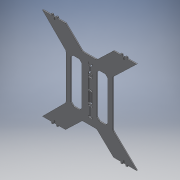
# Autodesk Inventor part: Z stage_brace
Saved by Autodesk Inventor 2019 (Build 230136000, 136)
## iProperties
Created: 2020-03-07
Part Number: Z stage_brace
Material: Generic
Document SubType Name: Modeling
Designer: Vijay
Density: 1 g/cm^3
Appearance: Default
Author: Vijay
Autodesk Inventor part; units mm, degrees
ref_plane "YZ Plane" through (0, 0, 0) normal (1, 0, 0) x (0, 1, 0)
ref_plane "XZ Plane" through (0, 0, 0) normal (0, 1, 0) x (-1, 0, 0)
ref_plane "XY Plane" through (0, 0, 0) normal (0, 0, 1) x (1, 0, 0)
sketch "Sketch1" plane through (0, 0, 0) normal (0, 0, 1) x (1, 0, 0)
  line L0 (428.5825, 0) -> (20, 0) projected
  line L1 (20, -400) -> (428.5825, -400) projected
  line L2 (328.5883, 0) -> (224.2968, -100)
  line L3 (224.2968, -100) -> (120, 0)
  line L4 (328.5825, -400) -> (224.2968, -300)
  line L5 (224.2968, -300) -> (120, -400)
  line L6 (224.2968, 24.0361) -> (224.2968, -493.2268) construction
  line L7 (428.5825, 0) -> (328.5883, 0)
  line L8 (120, 0) -> (19.9984, 0)
  line L9 (20, -400) -> (120, -400)
  line L10 (328.5825, -400) -> (428.5824, -400)
  line L11 (19.9984, 0) -> (122.1697, -102.1708)
  line L12 (122.1697, -102.1708) -> (122.1708, -297.8287)
  line L13 (122.1708, -297.8287) -> (20, -400)
  line L14 (428.5825, 0) -> (324.2968, -100.0061)
  line L15 (324.2968, -100.0061) -> (324.2968, -300)
  line L16 (324.2968, -300) -> (428.5824, -400)
  line L17 (255.5843, -70) -> (193.0078, -70)
  line L18 (255.5825, -330) -> (193.0078, -330)
  line L19 (20, -400) -> (20, -400)
  point P0 (0, 0)
  dimension "d1" = 100
  dimension "d2" = 100
  dimension "d3" = 100
  dimension "d4" = 104.2915
  dimension "d5" = 100
  dimension "d6" = 100
  dimension "d7" = 100
  dimension "d8" = 70
  dimension "d9" = 70
  constraints: 36 end point, 7 point on line, 4 equal length, 4 horizontal, 4 parallel, 3 perpendicular, 2 collinear, 2 vertical
  measures "d1" distance of L4.start L1.end
  measures "d2" distance of L5.end L1.start
  measures "d3" distance of L3.end L0.end
  measures "d4" distance from line of L6 L2.start
  measures "d5" distance from line of L0 L2.end
  measures "d6" distance from line of L1 L4.end
  measures "d7" distance between parallel lines of L6 L15
  measures "d8" distance between parallel lines of L0 L17
  measures "d9" distance between parallel lines of L1 L18
extrude "Extrusion1" add sketch "Sketch1" against normal blind 4 contours L14 L15 L16 L1 L4 L5 L13 L12 L11 L0 L3 L2 | L2 L3 L17 | L18 L5 L4
fillet "Fillet1" radius 10 8 edges at (324.2968, -100.0061, -2) (324.2968, -300, -2) (255.5825, -330, -2) (193.0078, -330, -2) (122.1708, -297.8287, -2) (122.1697, -102.1708, -2) (193.0078, -70, -2) (255.5843, -70, -2)
sketch "Sketch2" plane through (0, 0, -4) normal (0, 0, -1) x (-1, 0, 0)
  line L0 (-235.5222, -304.8491) -> (-235.5222, -94.8768) construction
  line L1 (-235.5222, -94.8768) -> (-217.757, -94.8768) construction
  line L2 (-217.757, -94.8768) -> (-217.757, -304.8491) construction
  line L3 (-217.757, -304.8491) -> (-235.5222, -304.8491) construction
  line L4 (-217.757, -297.1164) -> (-224.4247, -297.1164)
  line L5 (-224.4247, -297.1164) -> (-224.4247, -260.8142)
  line L6 (-224.4247, -260.8142) -> (-217.757, -260.8142)
  line L7 (-217.757, -260.8142) -> (-217.757, -255.0571)
  line L8 (-217.757, -255.0571) -> (-235.5222, -255.0571)
  line L9 (-235.5222, -255.0571) -> (-235.5222, -260.8142)
  line L10 (-235.5222, -260.8142) -> (-228.8545, -260.8142)
  line L11 (-228.8545, -260.8142) -> (-228.8545, -297.1164)
  line L12 (-228.8545, -297.1164) -> (-235.5222, -297.1164)
  line L13 (-235.5222, -297.1164) -> (-235.5222, -302.8735)
  line L14 (-235.5222, -302.8735) -> (-217.757, -302.8735)
  line L15 (-217.757, -302.8735) -> (-217.757, -297.1164)
  line L16 (-224.4247, -205.5429) -> (-228.8545, -205.5429)
  line L17 (-228.8545, -205.5429) -> (-228.8545, -245.3487)
  line L18 (-228.8545, -245.3487) -> (-229.7651, -245.3487)
  spline S0 degree 2 poles (-229.7651, -245.3487) (-230.3053, -245.3487) (-231.1079, -244.7777) (-231.1079, -244.1603) knots 0 0 0 1 2 2 2
  line L19 (-231.1079, -244.1603) -> (-231.1079, -205.4966)
  line L20 (-231.1079, -205.4966) -> (-235.5222, -205.4966)
  line L21 (-235.5222, -205.4966) -> (-235.5222, -247.17)
  spline S1 degree 2 poles (-235.5222, -247.17) (-235.5222, -249.2383) (-233.3923, -251.1058) (-231.5555, -251.1058) knots 0 0 0 1 2 2 2
  line L22 (-231.5555, -251.1058) -> (-221.7237, -251.1058)
  spline S2 degree 2 poles (-221.7237, -251.1058) (-219.887, -251.1058) (-217.757, -249.2383) (-217.757, -247.17) knots 0 0 0 1 2 2 2
  line L23 (-217.757, -247.17) -> (-217.757, -205.4966)
  line L24 (-217.757, -205.4966) -> (-222.1867, -205.4966)
  line L25 (-222.1867, -205.4966) -> (-222.1867, -244.1603)
  spline S3 degree 2 poles (-222.1867, -244.1603) (-222.1867, -244.7777) (-222.9739, -245.3487) (-223.5141, -245.3487) knots 0 0 0 1 2 2 2
  line L26 (-223.5141, -245.3487) -> (-224.4247, -245.3487)
  line L27 (-224.4247, -245.3487) -> (-224.4247, -205.5429)
  line L28 (-235.5222, -201.5453) -> (-221.7237, -201.5453)
  spline S4 degree 2 poles (-221.7237, -201.5453) (-219.887, -201.5453) (-217.757, -199.6778) (-217.757, -197.6095) knots 0 0 0 1 2 2 2
  line L29 (-217.757, -197.6095) -> (-217.757, -155.9361)
  line L30 (-217.757, -155.9361) -> (-222.1867, -155.9361)
  line L31 (-222.1867, -155.9361) -> (-222.1867, -194.5998)
  spline S5 degree 2 poles (-222.1867, -194.5998) (-222.1867, -195.2172) (-222.9739, -195.7882) (-223.5141, -195.7882) knots 0 0 0 1 2 2 2
  line L32 (-223.5141, -195.7882) -> (-235.5222, -195.7882)
  line L33 (-235.5222, -195.7882) -> (-235.5222, -201.5453)
  line L34 (-217.757, -146.1814) -> (-235.5222, -146.1814)
  line L35 (-235.5222, -146.1814) -> (-235.5222, -151.9848)
  line L36 (-235.5222, -151.9848) -> (-217.757, -151.9848)
  line L37 (-217.757, -151.9848) -> (-217.757, -146.1814)
  line L38 (-235.5222, -95.7103) -> (-235.5222, -103.3041)
  line L39 (-235.5222, -103.3041) -> (-228.8545, -111.4227)
  line L40 (-228.8545, -111.4227) -> (-228.8545, -127.6599)
  line L41 (-228.8545, -127.6599) -> (-235.5222, -135.7785)
  line L42 (-235.5222, -135.7785) -> (-235.5222, -143.3723)
  line L43 (-235.5222, -143.3723) -> (-226.6473, -132.7688)
  line L44 (-226.6473, -132.7688) -> (-217.757, -143.3723)
  line L45 (-217.757, -143.3723) -> (-217.757, -135.7785)
  line L46 (-217.757, -135.7785) -> (-224.4247, -127.6599)
  line L47 (-224.4247, -127.6599) -> (-224.4247, -111.4227)
  line L48 (-224.4247, -111.4227) -> (-217.757, -103.3041)
  line L49 (-217.757, -103.3041) -> (-217.757, -95.7103)
  line L50 (-217.757, -95.7103) -> (-226.6473, -106.3139)
  line L51 (-226.6473, -106.3139) -> (-235.5222, -95.7103)
  point P0 (0, 0)
  constraints: 2 other
extrude "Extrusion2" cut sketch "Sketch2" against normal blind 25.4
sketch "Sketch3" plane through (0, 0, 0) normal (0, 0, 1) x (1, 0, 0)
  line L0 (394.291, -17.6488) -> (394.291, 0) projected
  line L1 (394.291, 0) -> (387.4152, 0) projected
  line L2 (387.4152, 0) -> (387.4152, 6.35) projected
  line L3 (387.4152, 6.35) -> (381.4152, 6.35) projected
  line L4 (381.4152, 6.35) -> (381.4152, 0) projected
  line L5 (381.4152, 0) -> (375.3152, 0) projected
  line L6 (375.3152, 0) -> (375.3152, -6) projected
  line L7 (375.3152, -6) -> (376.5652, -6) projected
  line L8 (376.5652, -6) -> (376.5652, -8) projected
  line L9 (376.5652, -8) -> (375.3152, -8) projected
  line L10 (375.3152, -8) -> (375.3152, -10.65) projected
  line L11 (375.3152, -10.65) -> (372.3152, -10.65) projected
  line L12 (372.3152, -10.65) -> (372.3152, -8) projected
  line L13 (372.3152, -8) -> (371.0652, -8) projected
  line L14 (371.0652, -8) -> (371.0652, -6) projected
  line L15 (371.0652, -6) -> (372.3152, -6) projected
  line L16 (372.3152, -6) -> (372.3152, 0) projected
  line L17 (372.3152, 0) -> (366.2152, 0) projected
  line L18 (366.2152, 0) -> (366.2152, 6.35) projected
  line L19 (366.2152, 6.35) -> (360.2152, 6.35) projected
  line L20 (360.2152, 6.35) -> (360.2152, 0) projected
  line L21 (360.2152, 0) -> (353.3394, 0) projected
  line L22 (353.3394, 0) -> (353.3394, -17.6488) projected
  line L23 (353.3394, -17.6488) -> (394.291, -17.6488) projected
  line L24 (353.3404, -382.3505) -> (353.3405, -399.9993) projected
  line L25 (353.3405, -399.9993) -> (360.2163, -399.9992) projected
  line L26 (360.2163, -399.9992) -> (360.2164, -406.3492) projected
  line L27 (360.2164, -406.3492) -> (366.2164, -406.3492) projected
  line L28 (366.2164, -406.3492) -> (366.2163, -399.9992) projected
  line L29 (366.2163, -399.9992) -> (372.3163, -399.9992) projected
  line L30 (372.3163, -399.9992) -> (372.3163, -393.9992) projected
  line L31 (372.3163, -393.9992) -> (371.0663, -393.9992) projected
  line L32 (371.0663, -393.9992) -> (371.0663, -391.9992) projected
  line L33 (371.0663, -391.9992) -> (372.3163, -391.9992) projected
  line L34 (372.3163, -391.9992) -> (372.3163, -389.3492) projected
  line L35 (372.3163, -389.3492) -> (375.3163, -389.3491) projected
  line L36 (375.3163, -389.3491) -> (375.3163, -391.9991) projected
  line L37 (375.3163, -391.9991) -> (376.5663, -391.9991) projected
  line L38 (376.5663, -391.9991) -> (376.5663, -393.9991) projected
  line L39 (376.5663, -393.9991) -> (375.3163, -393.9991) projected
  line L40 (375.3163, -393.9991) -> (375.3163, -399.9991) projected
  line L41 (375.3163, -399.9991) -> (381.4163, -399.9991) projected
  line L42 (381.4163, -399.9991) -> (381.4164, -406.3491) projected
  line L43 (381.4164, -406.3491) -> (387.4164, -406.3491) projected
  line L44 (387.4164, -406.3491) -> (387.4163, -399.9991) projected
  line L45 (387.4163, -399.9991) -> (394.2922, -399.999) projected
  line L46 (394.2922, -399.999) -> (394.2921, -382.3503) projected
  line L47 (394.2921, -382.3503) -> (353.3404, -382.3505) projected
  line L48 (93.1211, -17.6495) -> (93.121, -0.0007) projected
  line L49 (93.121, -0.0007) -> (86.2452, -0.0008) projected
  line L50 (86.2452, -0.0008) -> (86.2452, 6.3492) projected
  line L51 (86.2452, 6.3492) -> (80.2452, 6.3492) projected
  line L52 (80.2452, 6.3492) -> (80.2452, -0.0008) projected
  line L53 (80.2452, -0.0008) -> (74.1452, -0.0009) projected
  line L54 (74.1452, -0.0009) -> (74.1452, -6.0009) projected
  line L55 (74.1452, -6.0009) -> (75.3952, -6.0008) projected
  line L56 (75.3952, -6.0008) -> (75.3952, -8.0008) projected
  line L57 (75.3952, -8.0008) -> (74.1452, -8.0009) projected
  line L58 (74.1452, -8.0009) -> (74.1453, -10.6509) projected
  line L59 (74.1453, -10.6509) -> (71.1453, -10.6509) projected
  line L60 (71.1453, -10.6509) -> (71.1453, -8.0009) projected
  line L61 (71.1453, -8.0009) -> (69.8953, -8.0009) projected
  line L62 (69.8953, -8.0009) -> (69.8952, -6.0009) projected
  line L63 (69.8952, -6.0009) -> (71.1452, -6.0009) projected
  line L64 (71.1452, -6.0009) -> (71.1452, -0.0009) projected
  line L65 (71.1452, -0.0009) -> (65.0452, -0.0009) projected
  line L66 (65.0452, -0.0009) -> (65.0452, 6.3491) projected
  line L67 (65.0452, 6.3491) -> (59.0452, 6.3491) projected
  line L68 (59.0452, 6.3491) -> (59.0452, -0.0009) projected
  line L69 (59.0452, -0.0009) -> (52.1694, -0.001) projected
  line L70 (52.1694, -0.001) -> (52.1695, -17.6498) projected
  line L71 (52.1695, -17.6498) -> (93.1211, -17.6495) projected
  line L72 (52.1715, -382.3522) -> (52.1716, -400.001) projected
  line L73 (52.1716, -400.001) -> (59.0475, -400.0009) projected
  line L74 (59.0475, -400.0009) -> (59.0475, -406.3509) projected
  line L75 (59.0475, -406.3509) -> (65.0475, -406.3509) projected
  line L76 (65.0475, -406.3509) -> (65.0475, -400.0009) projected
  line L77 (65.0475, -400.0009) -> (71.1475, -400.0009) projected
  line L78 (71.1475, -400.0009) -> (71.1474, -394.0009) projected
  line L79 (71.1474, -394.0009) -> (69.8974, -394.0009) projected
  line L80 (69.8974, -394.0009) -> (69.8974, -392.0009) projected
  line L81 (69.8974, -392.0009) -> (71.1474, -392.0009) projected
  line L82 (71.1474, -392.0009) -> (71.1474, -389.3509) projected
  line L83 (71.1474, -389.3509) -> (74.1474, -389.3509) projected
  line L84 (74.1474, -389.3509) -> (74.1474, -392.0009) projected
  line L85 (74.1474, -392.0009) -> (75.3974, -392.0008) projected
  line L86 (75.3974, -392.0008) -> (75.3974, -394.0008) projected
  line L87 (75.3974, -394.0008) -> (74.1474, -394.0009) projected
  line L88 (74.1474, -394.0009) -> (74.1475, -400.0009) projected
  line L89 (74.1475, -400.0009) -> (80.2475, -400.0008) projected
  line L90 (80.2475, -400.0008) -> (80.2475, -406.3508) projected
  line L91 (80.2475, -406.3508) -> (86.2475, -406.3508) projected
  line L92 (86.2475, -406.3508) -> (86.2475, -400.0008) projected
  line L93 (86.2475, -400.0008) -> (93.1233, -400.0007) projected
  line L94 (93.1233, -400.0007) -> (93.1232, -382.352) projected
  line L95 (93.1232, -382.352) -> (52.1715, -382.3522) projected
  point P0 (0, 0)
extrude "Extrusion3" add sketch "Sketch3" against normal up to surface (4 mm away)
sketch "Sketch4" plane through (0, 0, 0) normal (0, 0, 1) x (1, 0, 0)
  line L0 (394.291, -17.6488) -> (394.291, 0) projected
  line L1 (394.291, 0) -> (387.4152, 0) projected
  line L2 (387.4152, 0) -> (387.4152, 6.35) projected
  line L3 (387.4152, 6.35) -> (381.4152, 6.35) projected
  line L4 (381.4152, 6.35) -> (381.4152, 0) projected
  line L5 (381.4152, 0) -> (375.3152, 0) projected
  line L6 (375.3152, 0) -> (375.3152, -6) projected
  line L7 (375.3152, -6) -> (376.5652, -6) projected
  line L8 (376.5652, -6) -> (376.5652, -8) projected
  line L9 (376.5652, -8) -> (375.3152, -8) projected
  line L10 (375.3152, -8) -> (375.3152, -10.65) projected
  line L11 (375.3152, -10.65) -> (372.3152, -10.65) projected
  line L12 (372.3152, -10.65) -> (372.3152, -8) projected
  line L13 (372.3152, -8) -> (371.0652, -8) projected
  line L14 (371.0652, -8) -> (371.0652, -6) projected
  line L15 (371.0652, -6) -> (372.3152, -6) projected
  line L16 (372.3152, -6) -> (372.3152, 0) projected
  line L17 (372.3152, 0) -> (366.2152, 0) projected
  line L18 (366.2152, 0) -> (366.2152, 6.35) projected
  line L19 (366.2152, 6.35) -> (360.2152, 6.35) projected
  line L20 (360.2152, 6.35) -> (360.2152, 0) projected
  line L21 (360.2152, 0) -> (353.3394, 0) projected
  line L22 (353.3394, 0) -> (353.3394, -17.6488) projected
  line L23 (353.3394, -17.6488) -> (394.291, -17.6488) projected
  line L24 (353.3404, -382.3505) -> (353.3405, -399.9993) projected
  line L25 (353.3405, -399.9993) -> (360.2163, -399.9992) projected
  line L26 (360.2163, -399.9992) -> (360.2164, -406.3492) projected
  line L27 (360.2164, -406.3492) -> (366.2164, -406.3492) projected
  line L28 (366.2164, -406.3492) -> (366.2163, -400) projected
  line L29 (366.2163, -399.9992) -> (372.3163, -399.9992) projected
  line L30 (372.3163, -399.9992) -> (372.3163, -393.9992) projected
  line L31 (372.3163, -393.9992) -> (371.0663, -393.9992) projected
  line L32 (371.0663, -393.9992) -> (371.0663, -391.9992) projected
  line L33 (371.0663, -391.9992) -> (372.3163, -391.9992) projected
  line L34 (372.3163, -391.9992) -> (372.3163, -389.3492) projected
  line L35 (372.3163, -389.3492) -> (375.3163, -389.3491) projected
  line L36 (375.3163, -389.3491) -> (375.3163, -391.9991) projected
  line L37 (375.3163, -391.9991) -> (376.5663, -391.9991) projected
  line L38 (376.5663, -391.9991) -> (376.5663, -393.9991) projected
  line L39 (376.5663, -393.9991) -> (375.3163, -393.9991) projected
  line L40 (375.3163, -393.9991) -> (375.3163, -399.9991) projected
  line L41 (375.3163, -399.9991) -> (381.4163, -399.9991) projected
  line L42 (381.4163, -400) -> (381.4164, -406.3491) projected
  line L43 (381.4164, -406.3491) -> (387.4164, -406.3491) projected
  line L44 (387.4164, -406.3491) -> (387.4163, -399.9991) projected
  line L45 (387.4163, -399.9991) -> (394.2922, -399.999) projected
  line L46 (394.2922, -399.999) -> (394.2921, -382.3503) projected
  line L47 (394.2921, -382.3503) -> (353.3404, -382.3505) projected
  line L48 (52.1715, -382.3522) -> (52.1716, -400.001) projected
  line L49 (52.1716, -400.001) -> (59.0475, -400.0009) projected
  line L50 (59.0475, -400.0009) -> (59.0475, -406.3509) projected
  line L51 (59.0475, -406.3509) -> (65.0475, -406.3509) projected
  line L52 (65.0475, -406.3509) -> (65.0475, -400.0002) projected
  line L53 (93.1233, -400.0007) -> (71.1475, -400.0009) projected
  line L54 (71.1475, -400.0009) -> (71.1474, -394.0009) projected
  line L55 (71.1474, -394.0009) -> (69.8974, -394.0009) projected
  line L56 (69.8974, -394.0009) -> (69.8974, -392.0009) projected
  line L57 (69.8974, -392.0009) -> (71.1474, -392.0009) projected
  line L58 (71.1474, -392.0009) -> (71.1474, -389.3509) projected
  line L59 (71.1474, -389.3509) -> (74.1474, -389.3509) projected
  line L60 (74.1474, -389.3509) -> (74.1474, -392.0009) projected
  line L61 (74.1474, -392.0009) -> (75.3974, -392.0008) projected
  line L62 (75.3974, -392.0008) -> (75.3974, -394.0008) projected
  line L63 (75.3974, -394.0008) -> (74.1474, -394.0009) projected
  line L64 (74.1474, -394.0009) -> (74.1475, -400.0009) projected
  line L65 (74.1475, -400.0009) -> (120, -400.0006) projected
  line L66 (80.2475, -400.0002) -> (80.2475, -406.3508) projected
  line L67 (80.2475, -406.3508) -> (86.2475, -406.3508) projected
  line L68 (86.2475, -406.3508) -> (86.2475, -400.0008) projected
  line L69 (86.2475, -400.0008) -> (93.1233, -400.0007) projected
  line L70 (93.1233, -400.0007) -> (93.1232, -382.352) projected
  line L71 (93.1232, -382.352) -> (52.1715, -382.3522) projected
  line L72 (93.1211, -17.6495) -> (93.121, -0.0007) projected
  line L73 (93.121, -0.0007) -> (86.2452, -0.0008) projected
  line L74 (86.2452, -0.0008) -> (86.2452, 6.3492) projected
  line L75 (86.2452, 6.3492) -> (80.2452, 6.3492) projected
  line L76 (80.2452, 6.3492) -> (80.2452, 0) projected
  line L77 (80.2452, -0.0008) -> (74.1452, -0.0009) projected
  line L78 (74.1452, -0.0009) -> (74.1452, -6.0009) projected
  line L79 (74.1452, -6.0009) -> (75.3952, -6.0008) projected
  line L80 (75.3952, -6.0008) -> (75.3952, -8.0008) projected
  line L81 (75.3952, -8.0008) -> (74.1452, -8.0009) projected
  line L82 (74.1452, -8.0009) -> (74.1453, -10.6509) projected
  line L83 (74.1453, -10.6509) -> (71.1453, -10.6509) projected
  line L84 (71.1453, -10.6509) -> (71.1453, -8.0009) projected
  line L85 (71.1453, -8.0009) -> (69.8953, -8.0009) projected
  line L86 (69.8953, -8.0009) -> (69.8952, -6.0009) projected
  line L87 (69.8952, -6.0009) -> (71.1452, -6.0009) projected
  line L88 (71.1452, -6.0009) -> (71.1452, -0.0009) projected
  line L89 (71.1452, -0.0009) -> (65.0452, -0.0009) projected
  line L90 (65.0452, 0) -> (65.0452, 6.3491) projected
  line L91 (65.0452, 6.3491) -> (59.0452, 6.3491) projected
  line L92 (59.0452, 6.3491) -> (59.0452, -0.0009) projected
  line L93 (59.0452, -0.0009) -> (52.1694, -0.001) projected
  line L94 (52.1694, -0.001) -> (52.1695, -17.6498) projected
  line L95 (52.1695, -17.6498) -> (93.1211, -17.6495) projected
  line L96 (375.3152, 0) -> (372.3152, 0)
  line L97 (375.3163, -400) -> (372.3163, -400)
  line L98 (366.2163, -400) -> (381.4163, -400) projected
  line L99 (74.1475, -400) -> (71.1475, -400)
  line L100 (120, -400) -> (93.1233, -400) projected
  line L101 (74.1452, 0) -> (71.1452, 0)
  line L102 (65.0452, 0) -> (80.2452, 0) projected
  point P0 (0, 0)
  point P1 (93.1233, -400)
  point P2 (120, -400)
  constraints: 8 end point, 3 horizontal, 1 perpendicular, 3 other
extrude "Extrusion4" cut sketch "Sketch4" against normal blind 25.4 contours L6 L7 L8 L9 L10 L11 L12 L13 L14 L15 L16 L96 | L30 L31 L32 L33 L34 L35 L36 L37 L38 L39 L40 L97 | L53 L54 L55 L56 L57 L58 L59 L60 L61 L62 L63 L64 | L78 L79 L80 L81 L82 L83 L84 L85 L86 L87 L88 L101
sketch "Sketch5" plane through (0, 0, -4) normal (0, 0, -1) x (-1, 0, 0)
  line L0 (-228.8545, -111.4227) -> (-235.5222, -103.3041) projected
  line L1 (-235.5222, -103.3041) -> (-235.5222, -95.7103) projected
  line L2 (-235.5222, -95.7103) -> (-226.6473, -106.3139) projected
  line L3 (-226.6473, -106.3139) -> (-217.757, -95.7103) projected
  line L4 (-217.757, -95.7103) -> (-217.757, -103.3041) projected
  line L5 (-217.757, -103.3041) -> (-224.4247, -111.4227) projected
  line L6 (-224.4247, -111.4227) -> (-224.4247, -127.6599) projected
  line L7 (-224.4247, -127.6599) -> (-217.757, -135.7785) projected
  line L8 (-217.757, -135.7785) -> (-217.757, -143.3723) projected
  line L9 (-217.757, -143.3723) -> (-226.6473, -132.7688) projected
  line L10 (-226.6473, -132.7688) -> (-235.5222, -143.3723) projected
  line L11 (-235.5222, -143.3723) -> (-235.5222, -135.7785) projected
  line L12 (-235.5222, -135.7785) -> (-228.8545, -127.6599) projected
  line L13 (-228.8545, -127.6599) -> (-228.8545, -111.4227) projected
  line L14 (-221.7237, -201.5453) -> (-235.5222, -201.5453) projected
  line L15 (-235.5222, -201.5453) -> (-235.5222, -195.7882) projected
  line L16 (-235.5222, -195.7882) -> (-223.5141, -195.7882) projected
  line L17 (-222.1867, -194.5998) -> (-222.1867, -155.9361) projected
  line L18 (-222.1867, -155.9361) -> (-217.757, -155.9361) projected
  line L19 (-217.757, -155.9361) -> (-217.757, -197.6095) projected
  line L20 (-224.4247, -260.8142) -> (-224.4247, -297.1164) projected
  line L21 (-224.4247, -297.1164) -> (-217.757, -297.1164) projected
  line L22 (-217.757, -297.1164) -> (-217.757, -302.8735) projected
  line L23 (-217.757, -302.8735) -> (-235.5222, -302.8735) projected
  line L24 (-235.5222, -302.8735) -> (-235.5222, -297.1164) projected
  line L25 (-235.5222, -297.1164) -> (-228.8545, -297.1164) projected
  line L26 (-228.8545, -297.1164) -> (-228.8545, -260.8142) projected
  line L27 (-228.8545, -260.8142) -> (-235.5222, -260.8142) projected
  line L28 (-235.5222, -260.8142) -> (-235.5222, -255.0571) projected
  line L29 (-235.5222, -255.0571) -> (-217.757, -255.0571) projected
  line L30 (-217.757, -255.0571) -> (-217.757, -260.8142) projected
  line L31 (-217.757, -260.8142) -> (-224.4247, -260.8142) projected
  line L32 (-228.8545, -245.3487) -> (-228.8545, -205.5429) projected
  line L33 (-228.8545, -205.5429) -> (-224.4247, -205.5429) projected
  line L34 (-224.4247, -205.5429) -> (-224.4247, -245.3487) projected
  line L35 (-224.4247, -245.3487) -> (-223.5141, -245.3487) projected
  line L36 (-222.1867, -244.1603) -> (-222.1867, -205.4966) projected
  line L37 (-222.1867, -205.4966) -> (-217.757, -205.4966) projected
  line L38 (-217.757, -205.4966) -> (-217.757, -247.17) projected
  line L39 (-221.7237, -251.1058) -> (-231.5555, -251.1058) projected
  line L40 (-235.5222, -247.17) -> (-235.5222, -205.4966) projected
  line L41 (-235.5222, -205.4966) -> (-231.1079, -205.4966) projected
  line L42 (-231.1079, -205.4966) -> (-231.1079, -244.1603) projected
  line L43 (-229.7651, -245.3487) -> (-228.8545, -245.3487) projected
  line L44 (-235.5222, -151.9848) -> (-235.5222, -146.1814) projected
  line L45 (-235.5222, -146.1814) -> (-217.757, -146.1814) projected
  line L46 (-217.757, -146.1814) -> (-217.757, -151.9848) projected
  line L47 (-217.757, -151.9848) -> (-235.5222, -151.9848) projected
  line L48 (-71.1452, -0.0009) -> (-71.1452, -6.0009) projected
  line L49 (-71.1452, -6.0009) -> (-69.8952, -6.0009) projected
  line L50 (-69.8952, -6.0009) -> (-69.8953, -8.0009) projected
  line L51 (-69.8953, -8.0009) -> (-71.1453, -8.0009) projected
  line L52 (-71.1453, -8.0009) -> (-71.1453, -10.6509) projected
  line L53 (-71.1453, -10.6509) -> (-74.1453, -10.6509) projected
  line L54 (-74.1453, -10.6509) -> (-74.1452, -8.0009) projected
  line L55 (-74.1452, -8.0009) -> (-75.3952, -8.0008) projected
  line L56 (-75.3952, -8.0008) -> (-75.3952, -6.0008) projected
  line L57 (-75.3952, -6.0008) -> (-74.1452, -6.0009) projected
  line L58 (-74.1452, -6.0009) -> (-74.1452, -0.0009) projected
  line L59 (-74.1452, -0.0009) -> (-71.1452, -0.0009) projected
  line L60 (-375.3163, -399.9991) -> (-375.3163, -393.9991) projected
  line L61 (-375.3163, -393.9991) -> (-376.5663, -393.9991) projected
  line L62 (-376.5663, -393.9991) -> (-376.5663, -391.9991) projected
  line L63 (-376.5663, -391.9991) -> (-375.3163, -391.9991) projected
  line L64 (-375.3163, -391.9991) -> (-375.3163, -389.3491) projected
  line L65 (-375.3163, -389.3491) -> (-372.3163, -389.3492) projected
  line L66 (-372.3163, -389.3492) -> (-372.3163, -391.9992) projected
  line L67 (-372.3163, -391.9992) -> (-371.0663, -391.9992) projected
  line L68 (-371.0663, -391.9992) -> (-371.0663, -393.9992) projected
  line L69 (-371.0663, -393.9992) -> (-372.3163, -393.9992) projected
  line L70 (-372.3163, -393.9992) -> (-372.3163, -399.9992) projected
  line L71 (-372.3163, -399.9992) -> (-375.3163, -399.9991) projected
  line L72 (-74.1475, -400.0009) -> (-74.1474, -394.0009) projected
  line L73 (-74.1474, -394.0009) -> (-75.3974, -394.0008) projected
  line L74 (-75.3974, -394.0008) -> (-75.3974, -392.0008) projected
  line L75 (-75.3974, -392.0008) -> (-74.1474, -392.0009) projected
  line L76 (-74.1474, -392.0009) -> (-74.1474, -389.3509) projected
  line L77 (-74.1474, -389.3509) -> (-71.1474, -389.3509) projected
  line L78 (-71.1474, -389.3509) -> (-71.1474, -392.0009) projected
  line L79 (-71.1474, -392.0009) -> (-69.8974, -392.0009) projected
  line L80 (-69.8974, -392.0009) -> (-69.8974, -394.0009) projected
  line L81 (-69.8974, -394.0009) -> (-71.1474, -394.0009) projected
  line L82 (-71.1475, -400.0009) -> (-71.1474, -394.0009) projected
  line L83 (-65.0475, -400.0009) -> (-71.1475, -400.0009) projected
  line L84 (-65.0475, -406.3509) -> (-65.0475, -400.0009) projected
  line L85 (-59.0475, -406.3509) -> (-65.0475, -406.3509) projected
  line L86 (-59.0475, -400.0009) -> (-59.0475, -406.3509) projected
  line L87 (-52.1716, -400.001) -> (-59.0475, -400.0009) projected
  line L88 (-52.1716, -400) -> (-52.1716, -400.001) projected
  line L89 (-52.1716, -400) -> (-20, -400) projected
  line L90 (-20, -400) -> (-119.2418, -300.7577) projected
  arc A0 (-122.1707, -293.6866) -> (-119.2418, -300.7577) centre (-112.1707, -293.6866) ccw projected
  line L91 (-122.1707, -293.6866) -> (-122.1697, -106.3129) projected
  arc A1 (-119.2408, -99.2419) -> (-122.1697, -106.3129) centre (-112.1697, -106.313) ccw projected
  line L92 (-119.2408, -99.2419) -> (-19.9984, 0) projected
  line L93 (-19.9984, 0) -> (-59.0452, 0) projected
  line L94 (-59.0452, 6.3491) -> (-59.0452, 0) projected
  line L95 (-65.0452, 6.3491) -> (-59.0452, 6.3491) projected
  line L96 (-65.0452, 0) -> (-65.0452, 6.3491) projected
  line L97 (-65.0452, 0) -> (-80.2452, 0) projected
  line L98 (-80.2452, 6.3492) -> (-80.2452, 0) projected
  line L99 (-86.2452, 6.3492) -> (-80.2452, 6.3492) projected
  line L100 (-86.2452, 0) -> (-86.2452, 6.3492) projected
  line L101 (-86.2452, 0) -> (-120, 0) projected
  line L102 (-120, 0) -> (-190.1064, -67.2182) projected
  arc A2 (-197.0272, -70) -> (-190.1064, -67.2182) centre (-197.0272, -60) ccw projected
  line L103 (-197.0272, -70) -> (-251.5646, -70) projected
  arc A3 (-258.4856, -67.218) -> (-251.5646, -70) centre (-251.5646, -60) ccw projected
  line L104 (-258.4856, -67.218) -> (-328.5883, 0) projected
  line L105 (-328.5883, 0) -> (-360.2152, 0) projected
  line L106 (-360.2152, 6.35) -> (-360.2152, 0) projected
  line L107 (-366.2152, 6.35) -> (-360.2152, 6.35) projected
  line L108 (-366.2152, 0) -> (-366.2152, 6.35) projected
  line L109 (-366.2152, 0) -> (-372.3152, 0) projected
  line L110 (-372.3152, 0) -> (-372.3152, -6) projected
  line L111 (-372.3152, -6) -> (-371.0652, -6) projected
  line L112 (-371.0652, -6) -> (-371.0652, -8) projected
  line L113 (-371.0652, -8) -> (-372.3152, -8) projected
  line L114 (-372.3152, -8) -> (-372.3152, -10.65) projected
  line L115 (-372.3152, -10.65) -> (-375.3152, -10.65) projected
  line L116 (-375.3152, -10.65) -> (-375.3152, -8) projected
  line L117 (-375.3152, -8) -> (-376.5652, -8) projected
  line L118 (-376.5652, -8) -> (-376.5652, -6) projected
  line L119 (-376.5652, -6) -> (-375.3152, -6) projected
  line L120 (-375.3152, -6) -> (-375.3152, 0) projected
  line L121 (-375.3152, 0) -> (-381.4152, 0) projected
  line L122 (-381.4152, 6.35) -> (-381.4152, 0) projected
  line L123 (-387.4152, 6.35) -> (-381.4152, 6.35) projected
  line L124 (-387.4152, 0) -> (-387.4152, 6.35) projected
  line L125 (-387.4152, 0) -> (-428.5825, 0) projected
  line L126 (-428.5825, 0) -> (-327.3754, -97.0538) projected
  arc A4 (-324.2968, -104.2714) -> (-327.3754, -97.0538) centre (-334.2968, -104.2714) ccw projected
  line L127 (-324.2968, -104.2714) -> (-324.2968, -295.7344) projected
  arc A5 (-327.3756, -302.9522) -> (-324.2968, -295.7344) centre (-334.2968, -295.7344) ccw projected
  line L128 (-327.3756, -302.9522) -> (-428.5824, -400) projected
  line L129 (-428.5824, -400) -> (-387.4163, -400) projected
  line L130 (-387.4164, -406.3491) -> (-387.4163, -400) projected
  line L131 (-381.4164, -406.3491) -> (-387.4164, -406.3491) projected
  line L132 (-381.4163, -400) -> (-381.4164, -406.3491) projected
  line L133 (-381.4163, -400) -> (-366.2163, -400) projected
  line L134 (-366.2164, -406.3492) -> (-366.2163, -400) projected
  line L135 (-360.2164, -406.3492) -> (-366.2164, -406.3492) projected
  line L136 (-360.2163, -400) -> (-360.2164, -406.3492) projected
  line L137 (-360.2163, -400) -> (-328.5825, -400) projected
  line L138 (-328.5825, -400) -> (-258.4839, -332.7822) projected
  arc A6 (-251.5627, -330) -> (-258.4839, -332.7822) centre (-251.5627, -340) ccw projected
  line L139 (-251.5627, -330) -> (-197.0272, -330) projected
  arc A7 (-190.1064, -332.7818) -> (-197.0272, -330) centre (-197.0272, -340) ccw projected
  line L140 (-190.1064, -332.7818) -> (-120, -400) projected
  line L141 (-120, -400) -> (-93.1233, -400) projected
  line L142 (-93.1233, -400.0007) -> (-93.1233, -400) projected
  line L143 (-86.2475, -400.0008) -> (-93.1233, -400.0007) projected
  line L144 (-86.2475, -406.3508) -> (-86.2475, -400.0008) projected
  line L145 (-80.2475, -406.3508) -> (-86.2475, -406.3508) projected
  line L146 (-80.2475, -400.0008) -> (-80.2475, -406.3508) projected
  line L147 (-74.1475, -400.0009) -> (-80.2475, -400.0008) projected
  line L148 (-255.3002, -104.2714) -> (-304.2968, -104.2714)
  line L149 (-304.2968, -104.2714) -> (-304.2968, -295.7344)
  line L150 (-304.2968, -295.7344) -> (-255.3002, -295.7344)
  line L151 (-255.3002, -295.7344) -> (-255.3002, -104.2714)
  line L152 (-255.3002, -104.2714) -> (-304.2968, -295.7344) construction
  line L153 (-304.2968, -104.2714) -> (-255.3002, -295.7344) construction
  line L154 (-191.1674, -104.2714) -> (-142.1707, -104.2714)
  line L155 (-142.1707, -104.2714) -> (-142.1707, -295.7344)
  line L156 (-142.1707, -295.7344) -> (-191.1674, -295.7344)
  line L157 (-191.1674, -295.7344) -> (-191.1674, -104.2714)
  line L158 (-191.1674, -104.2714) -> (-142.1707, -295.7344) construction
  line L159 (-142.1707, -104.2714) -> (-191.1674, -295.7344) construction
  point P0 (0, 0)
  point P1 (-279.7985, -200.0029)
  point P2 (-166.669, -200.0029)
  dimension "d19" = 20
  dimension "d20" = 20
  constraints: 24 end point, 4 midpoint, 4 parallel, 3 collinear, 2 horizontal, 2 perpendicular, 2 point on line, 6 other
  measures "d19" distance between parallel lines of L149 L127
  measures "d20" horizontal distance of L91.start L155.end
extrude "Extrusion5" cut sketch "Sketch5" against normal through all contours L151 L150 L149 L148 | L154 L155 L156 L157
chamfer "Chamfer1" distance 11.1125 angle 45 8 edges at (304.2968, -295.7344, -2) (255.3002, -295.7344, -2) (255.3002, -104.2714, -2) (304.2968, -104.2714, -2) (191.1674, -295.7344, -2) (142.1707, -295.7344, -2) (142.1707, -104.2714, -2) (191.1674, -104.2714, -2)
body "Solid1"
